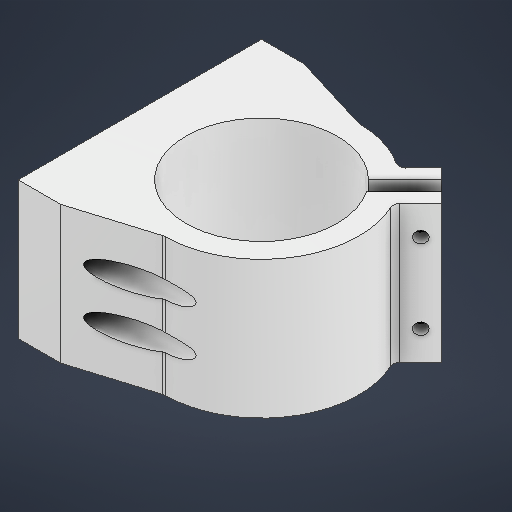
# Autodesk Inventor part: CNC-015-65mmSpindleMount
Saved by Autodesk Inventor 2026.2 (Build 302298000, 298)
## iProperties
Created: 2026-06-19
Part Number: CNC-015-65mmSpindleMount
Material: ABS Plastic
Document SubType Name: Modeling
Designer: Kenji
Density: 1.06 g/cm^3
Appearance: Smooth - White
Author: Kenji
Autodesk Inventor part; units mm, degrees
ref_plane "YZ Plane" through (0, 0, 0) normal (1, 0, 0) x (0, 1, 0)
ref_plane "XZ Plane" through (0, 0, 0) normal (0, 1, 0) x (-1, 0, 0)
ref_plane "XY Plane" through (0, 0, 0) normal (0, 0, 1) x (1, 0, 0)
sketch "Sketch1" plane through (0, 0, 0) normal (0, 1, 0) x (-1, 0, 0)
  circle A0 centre (0, 0) radius 32.5 construction
  arc A1 (-23.3345, -23.3345) -> (-27.3886, -18.4083) centre (0, 0) ccw
  line L0 (-27.3886, -18.4083) -> (-35.8094, -26.8292)
  line L1 (-23.3345, -23.3345) -> (-39.304, -39.304)
  line L2 (-31.3193, -31.3193) -> (-35.8094, -26.8292) construction
  line L3 (-33.5643, -29.0742) -> (-25.1161, -20.626) construction
  line L4 (0, 0) -> (0, -42.525) construction
  line L5 (-35.8094, -26.8292) -> (-43.7942, -34.8139)
  line L6 (-43.7942, -34.8139) -> (-48.2843, -30.3238)
  line L7 (-48.2843, -30.3238) -> (-39.1964, -21.2359)
  line L8 (-39.304, -39.304) -> (-34.8139, -43.7942)
  line L9 (-34.8139, -43.7942) -> (-27.0147, -35.9949)
  line L10 (0, 42.525) -> (52.05, 58.4383)
  line L11 (52.05, 58.4383) -> (52.05, -58.4383)
  line L12 (52.05, -58.4383) -> (0, -42.525)
  line L13 (0, 0) -> (33, 0) construction
  arc A2 (-23.2529, -35.6045) -> (0, -42.525) centre (0, 0) ccw
  arc A3 (0, 42.525) -> (-38.595, -17.855) centre (0, 0) ccw
  arc A4 (-39.1964, -21.2359) -> (-38.595, -17.855) centre (-41.3178, -19.1146) ccw
  arc A5 (-23.2529, -35.6045) -> (-27.0147, -35.9949) centre (-24.8933, -38.1162) ccw
  point P0 (-37.6777, -19.7172)
  point P1 (-25.2425, -34.2227)
  point P2 (42.525, 0)
  dimension "d0" = 65
  dimension "d1" = 0.5
  dimension "d3" = 6.35
  dimension "d4" = 45
  dimension "d5" = 6.35
  dimension "d8" = 15
  dimension "d9" = 17
  dimension "d10" = 9.525
  dimension "d11" = 9.525
  dimension "d12" = 9.525
  dimension "d13" = 3
  constraints: 29 end point, 13 point on circle, 5 centre point, 5 perpendicular, 5 point on line, 4 tangent, 3 midpoint, 2 coincident, 2 collinear, 2 equal length, 2 equal radius, 2 vertical, 1 horizontal, 1 horizontal alignment, 1 parallel, 3 other
  measures "d3" distance of L0.end L2.start
  measures "d4" angle of L3 L4
  measures "d5" distance between parallel lines of L7 L5
  measures "d8" distance of L6.end point (-37.678, -19.717)
  measures "d9" angle of L13 L12
  measures "d10" distance from line of point (42.525, 0) L11
  measures "d11" radial gap between concentric circles of A3 A1
  measures "d12" distance of L13.end point (42.525, 0)
  measures "d13" radius of A4
extrude "Extrusion1" add sketch "Sketch1" along normal blind 60
fillet "Fillet1" radius 4 2 edges at (0, 30, -42.525) (0, 30, 42.525)
sketch "Sketch2" plane through (-52.05, 0, -58.4383) normal (-1, 0, 0) x (0, 0, 1)
  line L0 (100.9596, 0) -> (100.9596, 60) projected
  line L1 (100.9596, 0) -> (40.5833, 0) projected
  line L2 (40.5833, 0) -> (40.5833, 60) projected
  line L3 (100.9596, 60) -> (40.5833, 60) projected
  line L4 (15.9169, 60) -> (15.9169, 0) projected
  line L5 (22.8338, 60) -> (15.9169, 60) projected
  line L6 (22.8338, 0) -> (22.8338, 60) projected
  line L7 (22.8338, 0) -> (15.9169, 0) projected
  circle A0 centre (12.7, 40) radius 2.6
  circle A1 centre (12.7, 20) radius 2.6
  circle A2 centre (104.1766, 40) radius 2.6
  circle A3 centre (104.1766, 20) radius 2.6
  line L8 (0, 0) -> (116.8766, 0) projected
  line L9 (0, 60) -> (116.8766, 60) projected
  line L10 (0, 0) -> (0, 60) projected
  line L11 (116.8766, 0) -> (116.8766, 60) projected
  point P0 (58.4383, 0)
  dimension "d17" = 5.2
  dimension "d18" = 60
  dimension "d19" = 20
  dimension "d20" = 20
  dimension "d21" = 12.7
  dimension "d22" = 12.7
  constraints: 4 centre point, 3 equal radius, 2 horizontal alignment, 2 vertical alignment
  measures "d17" diameter of A0
  measures "d18" distance between parallel lines of L8 L9
  measures "d19" distance from line of A2.centre L9
  measures "d20" distance from line of L8 A3.centre
  measures "d21" distance from line of A0.centre L10
  measures "d22" distance from line of L11 A2.centre
extrude "Extrusion2" cut sketch "Sketch2" against normal through all contours A0 | A1 | A2 | A3
ref_plane "Work Plane1" through (49.55, 0, -58.4383) normal (-1, 0, 0) x (0, 0, 1)
sketch "Sketch3" plane through (49.55, 0, -58.4383) normal (-1, 0, 0) x (0, 0, 1)
  circle A0 centre (104.1766, 40) radius 2.6 projected
  circle A1 centre (104.1766, 20) radius 2.6 projected
  circle A2 centre (12.7, 40) radius 2.6 projected
  circle A3 centre (12.7, 20) radius 2.6 projected
  circle A4 centre (12.7, 40) radius 5
  circle A5 centre (12.7, 20) radius 5
  circle A6 centre (104.1766, 40) radius 5
  circle A7 centre (104.1766, 20) radius 5
  point P0 (58.4383, 0)
  dimension "d26" = 10
  constraints: 4 centre point, 4 coincident, 3 equal radius
  measures "d26" diameter of A4
extrude "Extrusion3" cut sketch "Sketch3" along normal blind 92.075
sketch "Sketch4" plane through (48.2843, 0, -30.3238) normal (0.7071068, 0, 0.7071068) x (0.7071068, 0, -0.7071068)
  circle A0 centre (-6.4261, 47.3) radius 2.6
  line L0 (0, 0) -> (0, 60) projected
  line L1 (-12.8522, 0) -> (-12.8522, 60) projected
  line L2 (-12.8522, 60) -> (0, 60) projected
  circle A1 centre (-6.4261, 12.7) radius 2.6
  line L3 (-12.8522, 0) -> (0, 0) projected
  point P0 (-55.5843, 0)
  dimension "d29" = 5.2
  dimension "d30" = 12.8522
  dimension "d31" = 6.4261
  dimension "d32" = 12.7
  dimension "d33" = 12.7
  constraints: 2 centre point, 1 equal radius, 1 vertical alignment
  measures "d29" diameter of A0
  measures "d30" distance between parallel lines of L0 L1
  measures "d31" distance from line of A0.centre L1
  measures "d32" distance from line of A0.centre L2
  measures "d33" distance from line of L3 A1.centre
extrude "Extrusion4" cut sketch "Sketch4" against normal through all contours A0 | A1
sketch "Sketch5" plane through (27.0147, 0, -35.9949) normal (-0.7071068, 0, -0.7071068) x (-0.7071068, 0, 0.7071068)
  circle A0 centre (-4.6037, 47.3) radius 2.6 projected
  circle A1 centre (-4.6037, 12.7) radius 2.6 projected
  circle A2 centre (-4.6037, 47.3) radius 6
  circle A3 centre (-4.6037, 12.7) radius 6
  point P0 (44.5545, 0)
  dimension "d36" = 12
  constraints: 2 centre point, 2 coincident, 1 equal radius
  measures "d36" diameter of A2
extrude "Extrusion5" cut sketch "Sketch5" along normal blind 25.4
sketch "Sketch6" plane through (-52.05, 0, -58.4383) normal (-1, 0, 0) x (0, 0, 1)
  circle A0 centre (104.1766, 40) radius 2.6 projected
  circle A1 centre (12.7, 20) radius 2.6 projected
  circle A2 centre (104.1766, 20) radius 2.6 projected
  circle A3 centre (12.7, 40) radius 2.6 projected
  line L0 (0, 0) -> (116.8766, 0) projected
  line L1 (116.8766, 0) -> (116.8766, 60) projected
  line L2 (0, 60) -> (116.8766, 60) projected
  line L3 (0, 0) -> (0, 60) projected
  circle A4 centre (12.7, 40) radius 7.3625 construction
  circle A5 centre (12.7, 20) radius 5 projected
  circle A6 centre (12.7, 20) radius 7.3625 construction
  circle A7 centre (104.1766, 40) radius 7.3625 construction
  circle A8 centre (104.1766, 20) radius 7.3625 construction
  line L4 (5.3375, 60) -> (5.3375, 0)
  line L5 (111.5391, 60) -> (111.5391, 0)
  line L6 (0, 0) -> (116.8766, 0) projected
  point P0 (58.4383, 0)
  dimension "d39" = 4.7625
  constraints: 4 centre point, 4 end point, 4 point on line, 3 coincident, 3 equal radius, 2 perpendicular, 2 tangent
  measures "d39" radial gap between concentric circles of A4 A3
extrude "Extrusion6" cut sketch "Sketch6" against normal through all contours L3 L2 L4 L0 | L5 L2 L1 L0
sketch "Sketch7" plane through (-52.05, 0, -53.1008) normal (-1, 0, 0) x (0, 0, 1)
  line L0 (0, 60) -> (0, 0) projected
  line L1 (0, 0) -> (106.2016, 0) projected
  line L2 (106.2016, 0) -> (106.2016, 60) projected
  line L3 (0, 60) -> (106.2016, 60) projected
  circle A0 centre (98.8391, 40) radius 2.6 projected
  circle A1 centre (7.3625, 20) radius 2.6 projected
  circle A2 centre (98.8391, 20) radius 2.6 projected
  circle A3 centre (7.3625, 40) radius 2.6 projected
  point P0 (53.1008, 0)
extrude "Extrusion7" add sketch "Sketch7" along normal blind 1.0253
equation "\"d5\" = d3"
equation "\"d12\" = d11"
equation "\"d19\" = 0.333333 * d18"
equation "\"d20\" = d19"
equation "\"d22\" = d21"
equation "\"d31\" = 0.5 * d30"
equation "\"d33\" = d32"
body "Solid1"
